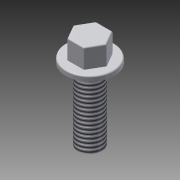
# Autodesk Inventor part: 载板下弹片固定螺丝
Saved by Autodesk Inventor 2015 (Build 190159000, 159)
## iProperties
Created: 2017-05-16
Part Number: 载板下弹片固定螺丝
Material: 常规
Document SubType Name: Modeling
Designer: Administrator
Density: 1 g/cm^3
Appearance: 雪
Author: Administrator
Autodesk Inventor part; units mm, degrees
ref_plane "YZ Plane" through (0, 0, 0) normal (1, 0, 0) x (0, 1, 0)
ref_plane "XZ Plane" through (0, 0, 0) normal (0, 1, 0) x (-1, 0, 0)
ref_plane "XY Plane" through (0, 0, 0) normal (0, 0, 1) x (1, 0, 0)
sketch "草图1" plane through (0, 0, 0) normal (0, 0, 1) x (1, 0, 0)
  circle A0 centre (0, 0) radius 5
  dimension "d0" = 10
  constraints: 1 centre point, 1 coincident
  measures "d0" diameter of A0
extrude "拉伸1" add sketch "草图1" along normal blind 5
sketch "草图2" plane through (0, 0, 5) normal (0, 0, 1) x (1, 0, 0)
  circle A0 centre (0, 0) radius 5
  circle A1 centre (0, 0) radius 5 projected
  line L0 (1.7321, -3) -> (-1.7321, -3)
  line L1 (-1.7321, -3) -> (-3.4641, 0)
  line L2 (-3.4641, 0) -> (-1.7321, 3)
  line L3 (-1.7321, 3) -> (1.7321, 3)
  line L4 (1.7321, 3) -> (3.4641, 0)
  line L5 (3.4641, 0) -> (1.7321, -3)
  line L6 (0, 0) -> (0, 1.0367)
  point P0 (0, 3)
  dimension "d3" = 1.0367
  dimension "d4" = 6
  constraints: 14 end point, 2 coincident, 2 concentric, 1 centre point, 1 midpoint, 1 point on line, 1 vertical, 13 other
  measures "d3" distance of L6.start L6.end
  measures "d4" distance between parallel lines of L0 L3
extrude "拉伸2" cut sketch "草图2" against normal blind 4
fillet "圆角1" radius 0.25 13 edges at (-5, 0, 1) (1.7321, 3, 3) (-2.5981, 1.5, 5) (0, 3, 5) (-1.7321, 3, 3) (-3.4641, 0, 3) (-2.5981, -1.5, 5) (-1.7321, -3, 3) (0, -3, 5) (2.5981, -1.5, 5) (1.7321, -3, 3) (3.4641, 0, 3) (2.5981, 1.5, 5)
sketch "草图3" plane through (0, 0, 0) normal (0, 0, -1) x (-1, 0, 0)
  circle A0 centre (0, 0) radius 2.5
  dimension "d8" = 5
  constraints: 1 centre point, 1 coincident
  measures "d8" diameter of A0
extrude "拉伸3" add sketch "草图3" along normal blind 15
thread "螺纹1" size "M5x0.8" class "6g" standard "ANSI Metric M Profile" full length
chamfer "倒角1" distance 0.225 angle 45 1 edges at (2.5, 0, -15)
